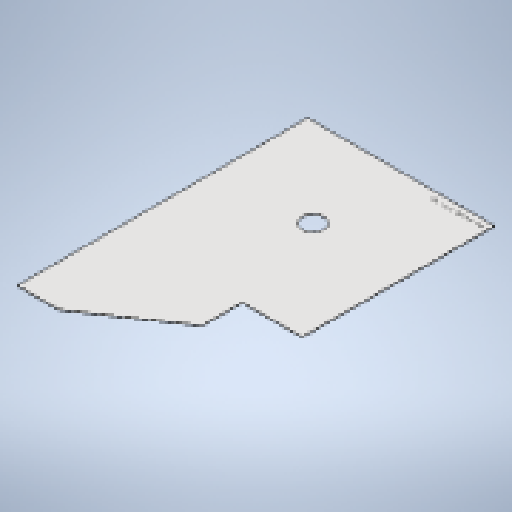
# Autodesk Inventor part: TRM 015 left board main
Saved by Autodesk Inventor 2025 (Build 290162010, 162A)
## iProperties
Created: 2024-08-07
Part Number: TRM 015 left board main
Material: AISI 304
Document SubType Name: Sheet Metal
Designer: pokla
Density: 8.02768 g/cm^3
Flat Pattern Width: 59.5257 cm
Flat Pattern Length: 105 cm
Flat Pattern Area: 6250.2 cm^2
Sheet Metal Rule: AISI304 2mm Die16
Sheet Metal Width: 595,257 mm
Sheet Metal Length: 1050,000 mm
Sheet Metal Area: 625019,533 mm^2
Appearance: Default
Stock Number: ТРМ 015 левый борт основное
Author: pokla
Autodesk Inventor part; units mm, degrees
ref_plane "YZ Plane" through (0, 0, 0) normal (1, 0, 0) x (0, 1, 0)
ref_plane "XZ Plane" through (0, 0, 0) normal (0, 1, 0) x (-1, 0, 0)
ref_plane "XY Plane" through (0, 0, 0) normal (0, 0, 1) x (1, 0, 0)
sketch "Sketch1" plane through (0, 0, 0) normal (0, 0, 1) x (1, 0, 0)
  line L0 (-319.0471, -452.819) -> (276.2096, -452.819)
  line L1 (276.2096, -452.819) -> (276.2096, 597.181)
  line L2 (276.2096, 597.181) -> (-319.0471, 597.181)
  line L3 (-319.0471, 597.181) -> (-319.0471, -452.819)
  line L4 (-78.0323, -452.819) -> (276.2096, 5.4517)
  circle A0 centre (0, 277.181) radius 40
  line L5 (276.2096, 5.4517) -> (176.2096, 5.4517)
  line L6 (176.2096, 5.4517) -> (176.2096, -123.9149)
  point P0 (0, 0)
  dimension "d1" = 1050
  dimension "d14" = 80
  dimension "d15" = 320
  dimension "d16" = 100
  measures "d1" distance of L1.end L0.end
  measures "d14" diameter of A0
  measures "d15" distance from line of A0.centre L2
  measures "d16" distance of L4.end L5.end
extrude "Plate1" add sketch "Sketch1" along normal blind 2 contours L3 L2 L1 L5 L6 L4 L0
sketch "Sketch2" plane through (0, 0, 0) normal (0, 0, -1) x (-1, 0, 0)
  line L0 (-256.2096, 577.181) -> (-56.2096, 577.181) construction
  line L1 (-56.2096, 577.181) -> (-56.2096, 557.181) construction
  line L2 (-56.2096, 557.181) -> (-256.2096, 557.181) construction
  line L3 (-256.2096, 557.181) -> (-256.2096, 577.181) construction
  line L4 (-276.2096, 597.181) -> (319.0471, 597.181) projected
  line L5 (-276.2096, 5.4517) -> (-276.2096, 597.181) projected
  point P0 (0, 0)
  point P1 (-48, 100)
  point P2 (-251, -525)
  point P3 (-50, 98)
  dimension "d6" = 200
  dimension "d9" = 20
  dimension "d10" = 20
  dimension "d11" = 20
  constraints: 4 other
  measures "d6" distance of L0.start L0.end
  measures "d9" distance of L0.end L1.end
  measures "d11" length of L3
mark "Mark1"
equation "\"d2\" = Thickness"
equation "\"BendReliefWidth\" = Thickness"
equation "\"BendReliefDepth\" = 0.5 * Thickness"
equation "\"CornerReliefSize\" = 4 * Thickness"
equation "\"MinimumRemnant\" = 2 * Thickness"
equation "\"TransitionRadius\" = BendRadius"
equation "\"JacobiRadiusSize\" = BendRadius"
equation "\"GapSize\" = Thickness"
equation "\"Thickness\" = 2"
equation "\"BendRadius\" = 2.75"
body "Solid1"
